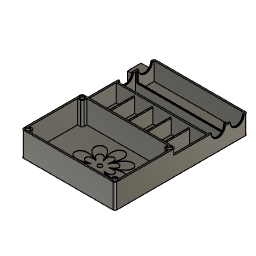
Wingspan - Nectar & Dice Container (Autodesk Fusion 360 design; units mm, degrees)
Autodesk Fusion 360 part; units mm, degrees
note: some values were not read from the file. Set by a fixed rule: which sketch regions a step uses.
sketch "Skizze1" plane through (0, 0, 0) normal (0, 0, 1) x (1, 0, 0)
  line L0 (0, 0) -> (107, 0)
  line L1 (107, 0) -> (107, 152)
  line L2 (107, 152) -> (0, 152)
  line L3 (0, 152) -> (0, 0)
  dimension "d1" = 107
  dimension "d2" = 152
  constraint horizontal L0
  constraint vertical L1
  constraint horizontal L2
  constraint vertical L3
  constraint coincident L0.start L3.end
  measures "d1" distance of L0.start L0.end
  measures "d2" distance of L0.start L2.end
extrude "Extrusion1" add sketch "Skizze1" against normal blind 28
sketch "Skizze2" plane through (0, 0, 0) normal (0, 0, 1) x (-1, 0, 0)
  line L0 (0, -152) -> (0, 0)
  line L1 (0, 0) -> (-107, 0)
  line L2 (-107, 0) -> (-107, -152)
  line L3 (-107, -152) -> (0, -152)
  line L4 (-1.75, -150.25) -> (-105.25, -150.25)
  line L5 (-105.25, -150.25) -> (-105.25, -130.25)
  line L6 (-105.25, -130.25) -> (-1.75, -130.25)
  line L7 (-1.75, -130.25) -> (-1.75, -150.25)
  line L8 (-105.25, -108.5) -> (-1.75, -108.5)
  line L9 (-1.75, -108.5) -> (-1.75, -128.5)
  line L10 (-1.75, -128.5) -> (-105.25, -128.5)
  line L11 (-105.25, -128.5) -> (-105.25, -108.5)
  dimension "d6" = 20
  dimension "d7" = 1.75
  dimension "d8" = 1.75
  dimension "d9" = 1.75
  dimension "d10" = 20
  dimension "d11" = 1.75
  dimension "d12" = 1.75
  dimension "d13" = 1.75
  constraint horizontal L4
  constraint vertical L5
  constraint horizontal L6
  constraint vertical L7
  constraint horizontal L10
  constraint vertical L11
  constraint horizontal L8
  constraint vertical L9
  measures "d6" distance of L4.start L6.end
  measures "d7" distance of L3 L4
  measures "d8" distance of L2 L5
  measures "d9" distance of L0 L7
  measures "d10" distance of L9.end L8.end
  measures "d11" distance of L6 L10
  measures "d12" distance of L2 L11
  measures "d13" distance of L0 L9
extrude "Extrusion2" cut sketch "Skizze2" against normal blind 27 contours L4 L5 L6 L7 | L8 L9 L10 L11
sketch "Skizze3" plane through (0, 0, 0) normal (0, 0, 1) x (-1, 0, 0)
  line L0 (-1.75, -108.5) -> (-1.75, -128.5)
  line L1 (-1.75, -128.5) -> (-105.25, -128.5)
  line L2 (-105.25, -128.5) -> (-105.25, -108.5)
  line L3 (-105.25, -108.5) -> (-1.75, -108.5)
  line L4 (-105.25, -150.25) -> (-105.25, -130.25)
  line L5 (-105.25, -130.25) -> (-1.75, -130.25)
  line L6 (-1.75, -130.25) -> (-1.75, -150.25)
  line L7 (-1.75, -150.25) -> (-105.25, -150.25)
  line L8 (0, -152) -> (0, 0)
  line L9 (0, 0) -> (-107, 0)
  line L10 (-107, 0) -> (-107, -152)
  line L11 (-107, -152) -> (0, -152)
  line L12 (0, -69.5) -> (-107, -69.5)
  dimension "d17" = 82.5
  constraint coincident L8 L12.start
  constraint coincident L10 L12.end
  constraint perpendicular L10 L12
  measures "d17" distance of L11 L12
extrude "Extrusion3" cut sketch "Skizze3" against normal blind 6.5 contours L8 L10 L11 L12
sketch "Skizze4" plane through (0, 0, -6.5) normal (0, 0, 1) x (-1, 0, 0)
  line L0 (-105.25, -128.5) -> (-105.25, -108.5)
  line L1 (-105.25, -108.5) -> (-1.75, -108.5)
  line L2 (-1.75, -108.5) -> (-1.75, -128.5)
  line L3 (-1.75, -128.5) -> (-105.25, -128.5)
  line L4 (-1.75, -130.25) -> (-1.75, -150.25)
  line L5 (-1.75, -150.25) -> (-105.25, -150.25)
  line L6 (-105.25, -150.25) -> (-105.25, -130.25)
  line L7 (-105.25, -130.25) -> (-1.75, -130.25)
  line L8 (0, -69.5) -> (-107, -69.5)
  line L9 (-107, -69.5) -> (-107, -152)
  line L10 (-107, -152) -> (0, -152)
  line L11 (0, -152) -> (0, -69.5)
  line L12 (-1.75, -106.75) -> (-105.25, -106.75)
  line L13 (-105.25, -106.75) -> (-105.25, -71.25)
  line L14 (-105.25, -71.25) -> (-1.75, -71.25)
  line L15 (-1.75, -71.25) -> (-1.75, -106.75)
  dimension "d21" = 1.75
  dimension "d22" = 1.75
  dimension "d23" = 1.75
  dimension "d24" = 1.75
  constraint horizontal L12
  constraint vertical L13
  constraint horizontal L14
  constraint vertical L15
  measures "d21" distance of L1 L12
  measures "d22" distance of L11 L15
  measures "d23" distance of L9 L13
  measures "d24" distance of L8 L14
extrude "Extrusion4" cut sketch "Skizze4" against normal blind 18 contours L12 L13 L14 L15
sketch "Skizze5" plane through (0, 0, -24.5) normal (0, 0, 1) x (-1, 0, 0)
  line L0 (-1.75, -71.25) -> (-105.25, -71.25)
  line L1 (-105.25, -71.25) -> (-105.25, -106.75)
  line L2 (-105.25, -106.75) -> (-1.75, -106.75)
  line L3 (-1.75, -106.75) -> (-1.75, -71.25)
  line L4 (-21.05, -106.75) -> (-22.8, -106.75)
  line L5 (-22.8, -106.75) -> (-22.8, -71.25)
  line L6 (-22.8, -71.25) -> (-21.05, -71.25)
  line L7 (-21.05, -71.25) -> (-21.05, -106.75)
  line L8 (-42.1, -106.75) -> (-43.85, -106.75)
  line L9 (-43.85, -106.75) -> (-43.85, -71.25)
  line L10 (-43.85, -71.25) -> (-42.1, -71.25)
  line L11 (-42.1, -71.25) -> (-42.1, -106.75)
  line L12 (-63.15, -106.75) -> (-64.9, -106.75)
  line L13 (-64.9, -106.75) -> (-64.9, -71.25)
  line L14 (-64.9, -71.25) -> (-63.15, -71.25)
  line L15 (-63.15, -71.25) -> (-63.15, -106.75)
  line L16 (-84.2, -106.75) -> (-85.95, -106.75)
  line L17 (-85.95, -106.75) -> (-85.95, -71.25)
  line L18 (-85.95, -71.25) -> (-84.2, -71.25)
  line L19 (-84.2, -71.25) -> (-84.2, -106.75)
  dimension "d27" = 1.75
  dimension "d28" = 1.75
  dimension "d29" = 1.75
  dimension "d30" = 1.75
  dimension "d31" = 19.3
  dimension "d32" = 19.3
  dimension "d33" = 19.3
  dimension "d34" = 19.3
  constraint horizontal L4
  constraint vertical L5
  constraint horizontal L6
  constraint vertical L7
  constraint coincident L0 L5.end
  constraint coincident L2 L4.start
  constraint horizontal L8
  constraint vertical L9
  constraint horizontal L10
  constraint vertical L11
  constraint coincident L0 L9.end
  constraint coincident L2 L8.start
  constraint horizontal L12
  constraint vertical L13
  constraint horizontal L14
  constraint vertical L15
  constraint coincident L0 L13.end
  constraint horizontal L16
  constraint vertical L17
  constraint horizontal L18
  constraint vertical L19
  constraint coincident L0 L17.end
  constraint coincident L2 L16.start
  measures "d27" distance of L5 L7
  measures "d28" distance of L9 L11
  measures "d29" distance of L13 L15
  measures "d30" distance of L17 L19
  measures "d31" distance of L3 L7
  measures "d32" distance of L5 L11
  measures "d33" distance of L9 L15
  measures "d34" distance of L13 L19
extrude "Extrusion5" add sketch "Skizze5" along normal blind 15 contours L0 L2 L4 L5 L6 L7 | L0 L2 L8 L9 L10 L11 | L0 L2 L12 L13 L14 L15 | L0 L2 L16 L17 L18 L19
sketch "Skizze6" plane through (0, 0, 0) normal (0, 0, 1) x (-1, 0, 0)
  line L0 (-107, -69.5) -> (0, -69.5)
  line L1 (0, -69.5) -> (0, 0)
  line L2 (0, 0) -> (-107, 0)
  line L3 (-107, 0) -> (-107, -69.5)
  line L4 (0, -69.5) -> (-7, -69.5)
  line L5 (-7, -69.5) -> (-7, -62.5)
  line L6 (-7, -62.5) -> (0, -62.5)
  line L7 (0, -62.5) -> (0, -69.5)
  line L8 (-107, -69.5) -> (-100, -69.5)
  line L9 (-100, -69.5) -> (-100, -62.5)
  line L10 (-100, -62.5) -> (-107, -62.5)
  line L11 (-107, -62.5) -> (-107, -69.5)
  line L12 (-107, 0) -> (-100, 0)
  line L13 (-100, 0) -> (-100, -7)
  line L14 (-100, -7) -> (-107, -7)
  line L15 (-107, -7) -> (-107, 0)
  line L16 (0, 0) -> (-7, 0)
  line L17 (-7, 0) -> (-7, -7)
  line L18 (-7, -7) -> (0, -7)
  line L19 (0, -7) -> (0, 0)
  circle A0 centre (-3.5, -3.5) radius 2.65
  circle A1 centre (-103.5, -3.5) radius 2.65
  circle A2 centre (-103.5, -66) radius 2.65
  circle A3 centre (-3.5, -66) radius 2.65
  line L20 (-7, -67.75) -> (-100, -67.75)
  line L21 (-100, -67.75) -> (-100, -1.75)
  line L22 (-100, -1.75) -> (-7, -1.75)
  line L23 (-7, -1.75) -> (-7, -67.75)
  line L24 (-7, -62.5) -> (-1.75, -62.5)
  line L25 (-1.75, -62.5) -> (-1.75, -7)
  line L26 (-1.75, -7) -> (-7, -7)
  line L27 (-7, -7) -> (-7, -62.5)
  line L28 (-100, -7) -> (-105.25, -7)
  line L29 (-105.25, -7) -> (-105.25, -62.5)
  line L30 (-105.25, -62.5) -> (-100, -62.5)
  line L31 (-100, -62.5) -> (-100, -7)
  dimension "d37" = 7
  dimension "d38" = 7
  dimension "d39" = 7
  dimension "d40" = 7
  dimension "d41" = 7
  dimension "d42" = 7
  dimension "d43" = 7
  dimension "d44" = 7
  dimension "d45" = 5.3
  dimension "d46" = 5.3
  dimension "d47" = 5.3
  dimension "d48" = 5.3
  dimension "d49" = 3.5
  dimension "d50" = 3.5
  dimension "d51" = 3.5
  dimension "d52" = 3.5
  dimension "d53" = 3.5
  dimension "d54" = 3.5
  dimension "d55" = 3.5
  dimension "d56" = 3.5
  dimension "d57" = 1.75
  dimension "d58" = 1.75
  dimension "d59" = 7
  dimension "d60" = 7
  dimension "d61" = 1.75
  dimension "d62" = 1.75
  constraint horizontal L4
  constraint vertical L5
  constraint horizontal L6
  constraint vertical L7
  constraint coincident L0.end L1.start
  constraint horizontal L8
  constraint vertical L9
  constraint horizontal L10
  constraint vertical L11
  constraint coincident L0.start L3.end
  constraint horizontal L12
  constraint vertical L13
  constraint horizontal L14
  constraint vertical L15
  constraint coincident L2.end L3.start
  constraint horizontal L16
  constraint vertical L17
  constraint horizontal L18
  constraint vertical L19
  constraint coincident L1.end L2.start
  constraint horizontal L20
  constraint vertical L21
  constraint horizontal L22
  constraint vertical L23
  constraint horizontal L24
  constraint vertical L25
  constraint horizontal L26
  constraint vertical L27
  constraint coincident L18 L25.end
  constraint horizontal L28
  constraint vertical L29
  constraint horizontal L30
  constraint vertical L31
  constraint coincident L10 L29.end
  measures "d37" distance of L0.end L4.end
  measures "d38" distance of L0.end L6.end
  measures "d39" distance of L0.start L8.end
  measures "d40" distance of L0.start L10.end
  measures "d41" distance of L2.end L12.end
  measures "d42" distance of L2.end L14.end
  measures "d43" distance of L1.end L16.end
  measures "d44" distance of L1.end L18.end
  measures "d45" diameter of A0
  measures "d46" diameter of A1
  measures "d47" diameter of A2
  measures "d48" diameter of A3
  measures "d49" distance of L7 A3.centre
  measures "d50" distance of L6 A3.centre
  measures "d51" distance of L10 A2.centre
  measures "d52" distance of L11 A2.centre
  measures "d53" distance of L15 A1.centre
  measures "d54" distance of L14 A1.centre
  measures "d55" distance of L18 A0.centre
  measures "d56" distance of L17 A0.centre
  measures "d57" distance of L0 L20
  measures "d58" distance of L2 L22
  measures "d59" distance of L1 L23
  measures "d60" distance of L3 L21
  measures "d61" distance of L1 L25
  measures "d62" distance of L3 L29
extrude "Extrusion6" cut sketch "Skizze6" against normal blind 26.25 contours L5 L9 L13 L17 L20 L21 L22 L23 L27 L31 | L10 L14 L21 L28 L29 L30 L31 | L6 L18 L23 L24 L25 L26 L27
extrude "Extrusion7" cut sketch "Skizze6" against normal blind 1.2 contours A0 | A1 | A2 | A3
sketch "Skizze7" plane through (0, 0, 0) normal (-1, 0, 0) x (0, -1, 0)
  line L0 (-69.5, 0) -> (-69.5, -6.5)
  line L1 (-69.5, -6.5) -> (-152, -6.5)
  line L2 (-152, -6.5) -> (-152, -28)
  line L3 (-152, -28) -> (0, -28)
  line L4 (0, -28) -> (0, 0)
  line L5 (0, 0) -> (-69.5, 0)
  line L6 (-152, -28) -> (-136.5, -28)
  line L7 (-136.5, -28) -> (-136.5, -18)
  line L8 (-136.5, -18) -> (-152, -18)
  line L9 (-152, -18) -> (-152, -28)
  dimension "d67" = 15.5
  dimension "d68" = 10
  constraint horizontal L6
  constraint vertical L7
  constraint horizontal L8
  constraint vertical L9
  constraint coincident L2.end L3.start
  measures "d67" distance of L2.end L6.end
  measures "d68" distance of L2.end L8.end
extrude "Extrusion8" add sketch "Skizze7" along normal blind 10 contours L2 L3 L6 L7 L8 L9
sketch "Skizze8" plane through (107, 0, 0) normal (1, 0, 0) x (0, 1, 0)
  line L0 (69.5, -6.5) -> (69.5, 0)
  line L1 (69.5, 0) -> (0, 0)
  line L2 (0, 0) -> (0, -28)
  line L3 (0, -28) -> (152, -28)
  line L4 (152, -28) -> (152, -6.5)
  line L5 (152, -6.5) -> (69.5, -6.5)
  circle A0 centre (140.25, -6.5) radius 7.5
  circle A1 centre (118.5, -6.5) radius 7.5
  dimension "d71" = 15
  dimension "d72" = 11.75
  dimension "d73" = 15
  dimension "d74" = 21.75
  constraint coincident L5 A0.centre
  constraint coincident L5 A1.centre
  measures "d71" diameter of A0
  measures "d72" distance of L4.end A0.centre
  measures "d73" diameter of A1
  measures "d74" distance of A0.centre A1.centre
extrude "Extrusion9" cut sketch "Skizze8" against normal blind 145 contours L5 A1 | L5 A0 picked at (120.0587, -9.1998) picked at (142.75, -10.4092)
extrude "Extrusion10" cut 1 faces at (-10, 146.8333, -24.6667) along direction (1, 0, 0) blind 10
sketch "Skizze9" plane through (0, 0, -6.5) normal (0, 0, 1) x (-1, 0, 0)
  line L0 (-107, -132.75) -> (-105.25, -132.75)
  line L1 (-105.25, -132.75) -> (-105.25, -130.25)
  line L2 (-105.25, -130.25) -> (-1.75, -130.25)
  line L3 (-1.75, -130.25) -> (-1.75, -132.75)
  line L4 (-1.75, -132.75) -> (0, -132.75)
  line L5 (0, -132.75) -> (0, -126)
  line L6 (0, -126) -> (-1.75, -126)
  line L7 (-1.75, -126) -> (-1.75, -128.5)
  line L8 (-1.75, -128.5) -> (-105.25, -128.5)
  line L9 (-105.25, -128.5) -> (-105.25, -126)
  line L10 (-105.25, -126) -> (-107, -126)
  line L11 (-107, -126) -> (-107, -132.75)
  line L12 (-4, -130.25) -> (-103, -130.25)
  line L13 (-103, -130.25) -> (-103, -128.5)
  line L14 (-103, -128.5) -> (-4, -128.5)
  line L15 (-4, -128.5) -> (-4, -130.25)
  dimension "d79" = 4
  dimension "d80" = 4
  constraint horizontal L12
  constraint vertical L13
  constraint horizontal L14
  constraint vertical L15
  constraint coincident L8 L13.end
  constraint coincident L2 L12.start
  measures "d79" distance of L5 L15
  measures "d80" distance of L11 L13
extrude "Extrusion11" cut sketch "Skizze9" against normal blind 10 contours L2 L8 L12 L13 L14 L15
extrude "Extrusion12" add sketch "Skizze7" along normal blind 15 contours L2 L3 L6 L7 L8 L9
fillet "Abrundung1" radius 2 6 edges at (0, 0, -14) (107, 0, -14) (7, 62.5, -13.125) (100, 62.5, -13.125) (100, 7, -13.125) (7, 7, -13.125)
fillet "Abrundung2" radius 2 2 edges at (107, 69.5, -3.25) (0, 69.5, -3.25)
fillet "Abrundung3" radius 2 2 edges at (107, 152, -17.25) (0, 152, -12.25)
fillet "Abrundung4" radius 0.5 2 edges at (53.5, 130.25, -16.5) (53.5, 128.5, -16.5)
fillet "Abrundung5" radius 0.75 8 edges at (22.8, 89, -9.5) (21.05, 89, -9.5) (43.85, 89, -9.5) (42.1, 89, -9.5) (64.9, 89, -9.5) (63.15, 89, -9.5) (85.95, 89, -9.5) (84.2, 89, -9.5)
sketch "Skizze10" plane through (0, 0, -26.25) normal (0, 0, 1) x (-1, 0, 0)
  line L0 (-102, -7) -> (-105.25, -7)
  line L1 (-105.25, -7) -> (-105.25, -62.5)
  line L2 (-105.25, -62.5) -> (-102, -62.5)
  arc A0 (-100, -64.5) -> (-102, -62.5) centre (-102, -64.5) ccw
  line L3 (-100, -64.5) -> (-100, -67.75)
  line L4 (-100, -67.75) -> (-7, -67.75)
  line L5 (-7, -67.75) -> (-7, -64.5)
  arc A1 (-5, -62.5) -> (-7, -64.5) centre (-5, -64.5) ccw
  line L6 (-5, -62.5) -> (-1.75, -62.5)
  line L7 (-1.75, -62.5) -> (-1.75, -7)
  line L8 (-1.75, -7) -> (-5, -7)
  arc A2 (-7, -5) -> (-5, -7) centre (-5, -5) ccw
  line L9 (-7, -5) -> (-7, -1.75)
  line L10 (-7, -1.75) -> (-100, -1.75)
  line L11 (-100, -1.75) -> (-100, -5)
  arc A3 (-102, -7) -> (-100, -5) centre (-102, -5) ccw
  spline S0 degree 3 poles (-56.5592, -62.8702) (-58.3493, -62.3021) (-60.0393, -60.5207) (-60.7133, -58.4915) knots 0 0 0 0 1 1 1 1
  spline S1 degree 3 poles (-60.7133, -58.4915) (-61.4989, -56.1264) (-61.1983, -52.2556) (-59.8935, -47.9352) knots 0 0 0 0 1 1 1 1
  spline S2 degree 3 poles (-59.8935, -47.9352) (-59.3339, -46.082) (-58.9465, -44.4517) (-59.0327, -44.3123) knots 0 0 0 0 1 1 1 1
  spline S3 degree 3 poles (-59.0327, -44.3123) (-59.1188, -44.1728) (-58.7988, -43.3306) (-58.3216, -42.4407) knots 0 0 0 0 1 1 1 1
  spline S4 degree 3 poles (-58.3216, -42.4407) (-57.8443, -41.5508) (-57.5275, -41.1269) (-57.6175, -41.4989) knots 0 0 0 0 1 1 1 1
  spline S5 degree 3 poles (-57.6175, -41.4989) (-57.7075, -41.8708) (-57.9588, -42.9002) (-58.176, -43.7864) knots 0 0 0 0 1 1 1 1
  spline S6 degree 3 poles (-58.176, -43.7864) (-58.3931, -44.6726) (-58.4995, -46.2578) (-58.4123, -47.309) knots 0 0 0 0 1 1 1 1
  spline S7 degree 3 poles (-58.4123, -47.309) (-58.2782, -48.9263) (-58.0889, -49.3677) (-57.1821, -50.178) knots 0 0 0 0 1 1 1 1
  spline S8 degree 3 poles (-57.1821, -50.178) (-55.6542, -51.5432) (-54.0418, -51.4908) (-52.5795, -50.0285) knots 0 0 0 0 1 1 1 1
  spline S9 degree 3 poles (-52.5795, -50.0285) (-50.8387, -48.2877) (-50.7558, -45.8848) (-52.2827, -41.4252) knots 0 0 0 0 1 1 1 1
  spline S10 degree 3 poles (-52.2827, -41.4252) (-52.3962, -41.0938) (-51.8778, -41.8116) (-51.1307, -43.0205) knots 0 0 0 0 1 1 1 1
  spline S11 degree 3 poles (-51.1307, -43.0205) (-49.292, -45.9958) (-47.7092, -47.2471) (-45.7844, -47.2471) knots 0 0 0 0 1 1 1 1
  spline S12 degree 3 poles (-45.7844, -47.2471) (-44.615, -47.2471) (-44.1039, -47.049) (-43.3644, -46.3095) knots 0 0 0 0 1 1 1 1
  spline S13 degree 3 poles (-43.3644, -46.3095) (-41.3829, -44.328) (-42.4992, -41.0532) (-45.8196, -39.1074) knots 0 0 0 0 1 1 1 1
  spline S14 degree 3 poles (-45.8196, -39.1074) (-47.2511, -38.2685) (-47.7575, -37.6104) (-46.9716, -37.6104) knots 0 0 0 0 1 1 1 1
  spline S15 degree 3 poles (-46.9716, -37.6104) (-46.7747, -37.6104) (-46.6847, -37.7256) (-46.7717, -37.8663) knots 0 0 0 0 1 1 1 1
  spline S16 degree 3 poles (-46.7717, -37.8663) (-46.8587, -38.0071) (-45.801, -38.1656) (-44.4211, -38.2186) knots 0 0 0 0 1 1 1 1
  spline S17 degree 3 poles (-44.4211, -38.2186) (-41.4525, -38.3326) (-39.7946, -37.7064) (-39.0007, -36.1712) knots 0 0 0 0 1 1 1 1
  spline S18 degree 3 poles (-39.0007, -36.1712) (-37.9053, -34.053) (-39.4569, -31.4883) (-42.138, -30.9853) knots 0 0 0 0 1 1 1 1
  spline S19 degree 3 poles (-42.138, -30.9853) (-43.1628, -30.7931) (-45.7249, -31.1569) (-47.6678, -31.7705) knots 0 0 0 0 1 1 1 1
  spline S20 degree 3 poles (-47.6678, -31.7705) (-47.9468, -31.8586) (-47.2483, -31.3259) (-46.1157, -30.5867) knots 0 0 0 0 1 1 1 1
  spline S21 degree 3 poles (-46.1157, -30.5867) (-43.7478, -29.0412) (-42.5959, -27.4189) (-42.5959, -25.6292) knots 0 0 0 0 1 1 1 1
  spline S22 degree 3 poles (-42.5959, -25.6292) (-42.5959, -23.9375) (-43.1044, -23.1064) (-44.4952, -22.5253) knots 0 0 0 0 1 1 1 1
  spline S23 degree 3 poles (-44.4952, -22.5253) (-46.2045, -21.8111) (-47.9424, -22.3756) (-49.568, -24.173) knots 0 0 0 0 1 1 1 1
  spline S24 degree 3 poles (-49.568, -24.173) (-50.2812, -24.9616) (-50.9936, -25.565) (-51.1511, -25.5139) knots 0 0 0 0 1 1 1 1
  spline S25 degree 3 poles (-51.1511, -25.5139) (-51.3086, -25.4628) (-51.3439, -25.5725) (-51.2295, -25.7576) knots 0 0 0 0 1 1 1 1
  spline S26 degree 3 poles (-51.2295, -25.7576) (-51.021, -26.0949) (-51.9974, -28.3217) (-52.2451, -28.0739) knots 0 0 0 0 1 1 1 1
  spline S27 degree 3 poles (-52.2451, -28.0739) (-52.3176, -28.0015) (-52.1542, -27.2023) (-51.882, -26.2981) knots 0 0 0 0 1 1 1 1
  spline S28 degree 3 poles (-51.882, -26.2981) (-50.8258, -22.7886) (-51.5141, -19.8497) (-53.6271, -18.847) knots 0 0 0 0 1 1 1 1
  spline S29 degree 3 poles (-53.6271, -18.847) (-55.6301, -17.8965) (-57.5857, -18.8268) (-58.4654, -21.1486) knots 0 0 0 0 1 1 1 1
  spline S30 degree 3 poles (-58.4654, -21.1486) (-59.0459, -22.6806) (-58.7942, -24.8474) (-57.6334, -28.3119) knots 0 0 0 0 1 1 1 1
  spline S31 degree 3 poles (-57.6334, -28.3119) (-57.5088, -28.6838) (-57.8962, -28.1512) (-58.4944, -27.1284) knots 0 0 0 0 1 1 1 1
  spline S32 degree 3 poles (-58.4944, -27.1284) (-60.4538, -23.778) (-62.1707, -22.3946) (-64.3696, -22.3946) knots 0 0 0 0 1 1 1 1
  spline S33 degree 3 poles (-64.3696, -22.3946) (-68.1521, -22.3946) (-68.6377, -27.3285) (-65.1088, -29.9052) knots 0 0 0 0 1 1 1 1
  spline S34 degree 3 poles (-65.1088, -29.9052) (-64.3499, -30.4593) (-63.7732, -31.0689) (-63.8273, -31.2599) knots 0 0 0 0 1 1 1 1
  spline S35 degree 3 poles (-63.8273, -31.2599) (-63.8847, -31.4625) (-63.6735, -31.511) (-63.3201, -31.3765) knots 0 0 0 0 1 1 1 1
  spline S36 degree 3 poles (-63.3201, -31.3765) (-62.9224, -31.225) (-62.8306, -31.2596) (-63.0527, -31.4773) knots 0 0 0 0 1 1 1 1
  spline S37 degree 3 poles (-63.0527, -31.4773) (-63.2735, -31.6937) (-63.983, -31.6897) (-65.098, -31.4659) knots 0 0 0 0 1 1 1 1
  spline S38 degree 3 poles (-65.098, -31.4659) (-68.378, -30.8075) (-71.3368, -32.4955) (-71.3368, -35.0251) knots 0 0 0 0 1 1 1 1
  spline S39 degree 3 poles (-71.3368, -35.0251) (-71.3368, -38.0388) (-67.7534, -39.4474) (-63.4113, -38.1407) knots 0 0 0 0 1 1 1 1
  spline S40 degree 3 poles (-63.4113, -38.1407) (-61.5097, -37.5684) (-61.5064, -37.5632) (-64.1235, -39.2548) knots 0 0 0 0 1 1 1 1
  spline S41 degree 3 poles (-64.1235, -39.2548) (-67.6237, -41.5171) (-68.5135, -44.6269) (-66.2141, -46.5617) knots 0 0 0 0 1 1 1 1
  spline S42 degree 3 poles (-66.2141, -46.5617) (-64.4839, -48.0175) (-61.8719, -47.4084) (-59.9372, -45.0979) knots 0 0 0 0 1 1 1 1
  spline S43 degree 3 poles (-59.9372, -45.0979) (-59.5254, -44.6062) (-59.1831, -44.3384) (-59.1764, -44.5028) knots 0 0 0 0 1 1 1 1
  spline S44 degree 3 poles (-59.1764, -44.5028) (-59.1603, -44.8983) (-61.7652, -50.0133) (-62.6404, -51.3046) knots 0 0 0 0 1 1 1 1
  spline S45 degree 3 poles (-62.6404, -51.3046) (-64.8787, -54.6074) (-67.8698, -56.5364) (-70.7619, -56.5423) knots 0 0 0 0 1 1 1 1
  spline S46 degree 3 poles (-70.7619, -56.5423) (-74.6622, -56.5503) (-77.4468, -52.9616) (-76.4404, -49.2242) knots 0 0 0 0 1 1 1 1
  spline S47 degree 3 poles (-76.4404, -49.2242) (-75.5977, -46.0946) (-73.3487, -43.7833) (-68.2937, -40.8517) knots 0 0 0 0 1 1 1 1
  spline S48 degree 3 poles (-68.2937, -40.8517) (-67.0849, -40.1506) (-66.4002, -39.6772) (-66.7721, -39.7996) knots 0 0 0 0 1 1 1 1
  spline S49 degree 3 poles (-66.7721, -39.7996) (-69.2344, -40.6101) (-74.0069, -41.6679) (-75.201, -41.6679) knots 0 0 0 0 1 1 1 1
  spline S50 degree 3 poles (-75.201, -41.6679) (-78.3788, -41.6679) (-81.566, -40.0721) (-82.6763, -37.925) knots 0 0 0 0 1 1 1 1
  spline S51 degree 3 poles (-82.6763, -37.925) (-83.3903, -36.5444) (-83.3099, -33.6152) (-82.5226, -32.324) knots 0 0 0 0 1 1 1 1
  spline S52 degree 3 poles (-82.5226, -32.324) (-81.7029, -30.9798) (-79.9968, -29.6996) (-78.2996, -29.1552) knots 0 0 0 0 1 1 1 1
  spline S53 degree 3 poles (-78.2996, -29.1552) (-76.383, -28.5404) (-71.7514, -28.9223) (-68.2937, -29.9801) knots 0 0 0 0 1 1 1 1
  spline S54 degree 3 poles (-68.2937, -29.9801) (-66.7129, -30.4637) (-65.1153, -30.9414) (-64.7433, -31.0416) knots 0 0 0 0 1 1 1 1
  spline S55 degree 3 poles (-64.7433, -31.0416) (-64.3714, -31.1419) (-65.6092, -30.4005) (-67.4941, -29.3941) knots 0 0 0 0 1 1 1 1
  spline S56 degree 3 poles (-67.4941, -29.3941) (-72.2017, -26.8806) (-73.8514, -25.6231) (-75.3197, -23.4291) knots 0 0 0 0 1 1 1 1
  spline S57 degree 3 poles (-75.3197, -23.4291) (-76.4762, -21.7011) (-76.5778, -21.356) (-76.5778, -19.1561) knots 0 0 0 0 1 1 1 1
  spline S58 degree 3 poles (-76.5778, -19.1561) (-76.5778, -17.0784) (-76.4577, -16.6054) (-75.6671, -15.5688) knots 0 0 0 0 1 1 1 1
  spline S59 degree 3 poles (-75.6671, -15.5688) (-73.5767, -12.8281) (-69.7646, -12.4778) (-66.4998, -14.7263) knots 0 0 0 0 1 1 1 1
  spline S60 degree 3 poles (-66.4998, -14.7263) (-64.4837, -16.1149) (-63.2894, -17.6345) (-60.7914, -21.9893) knots 0 0 0 0 1 1 1 1
  spline S61 degree 3 poles (-60.7914, -21.9893) (-59.8635, -23.607) (-59.1786, -24.6915) (-59.2695, -24.3993) knots 0 0 0 0 1 1 1 1
  spline S62 degree 3 poles (-59.2695, -24.3993) (-59.3604, -24.1071) (-59.8438, -22.5855) (-60.3437, -21.018) knots 0 0 0 0 1 1 1 1
  spline S63 degree 3 poles (-60.3437, -21.018) (-61.4281, -17.6182) (-61.7986, -13.6027) (-61.2022, -11.7145) knots 0 0 0 0 1 1 1 1
  spline S64 degree 3 poles (-61.2022, -11.7145) (-59.817, -7.3289) (-55.9762, -5.3552) (-52.3885, -7.1855) knots 0 0 0 0 1 1 1 1
  spline S65 degree 3 poles (-52.3885, -7.1855) (-48.7171, -9.0585) (-47.7733, -14.2699) (-49.879, -21.0421) knots 0 0 0 0 1 1 1 1
  spline S66 degree 3 poles (-49.879, -21.0421) (-51.2433, -25.4298) (-51.2167, -25.5019) (-49.4657, -22.1589) knots 0 0 0 0 1 1 1 1
  spline S67 degree 3 poles (-49.4657, -22.1589) (-47.2727, -17.9721) (-45.9857, -16.2284) (-44.052, -14.8244) knots 0 0 0 0 1 1 1 1
  spline S68 degree 3 poles (-44.052, -14.8244) (-41.0966, -12.6788) (-38.3228, -12.4229) (-35.8388, -14.0667) knots 0 0 0 0 1 1 1 1
  spline S69 degree 3 poles (-35.8388, -14.0667) (-32.6466, -16.1792) (-32.583, -20.6998) (-35.6935, -24.3965) knots 0 0 0 0 1 1 1 1
  spline S70 degree 3 poles (-35.6935, -24.3965) (-36.7851, -25.6938) (-39.6299, -27.663) (-42.5114, -29.1158) knots 0 0 0 0 1 1 1 1
  spline S71 degree 3 poles (-42.5114, -29.1158) (-43.6737, -29.7018) (-44.6247, -30.2455) (-44.6247, -30.3241) knots 0 0 0 0 1 1 1 1
  spline S72 degree 3 poles (-44.6247, -30.3241) (-44.6247, -30.4026) (-43.2933, -30.0073) (-41.6661, -29.4456) knots 0 0 0 0 1 1 1 1
  spline S73 degree 3 poles (-41.6661, -29.4456) (-37.8603, -28.132) (-33.6642, -27.7981) (-31.2092, -28.6136) knots 0 0 0 0 1 1 1 1
  spline S74 degree 3 poles (-31.2092, -28.6136) (-25.6033, -30.4756) (-25.0764, -37.2838) (-30.3383, -39.8677) knots 0 0 0 0 1 1 1 1
  spline S75 degree 3 poles (-30.3383, -39.8677) (-33.0905, -41.2191) (-36.6516, -41.1596) (-41.4863, -39.6813) knots 0 0 0 0 1 1 1 1
  spline S76 degree 3 poles (-41.4863, -39.6813) (-43.3866, -39.1002) (-45.0603, -38.6277) (-45.2057, -38.6313) knots 0 0 0 0 1 1 1 1
  spline S77 degree 3 poles (-45.2057, -38.6313) (-45.3511, -38.6349) (-44.0838, -39.3737) (-42.3896, -40.2731) knots 0 0 0 0 1 1 1 1
  spline S78 degree 3 poles (-42.3896, -40.2731) (-36.727, -43.2794) (-35.2415, -44.5962) (-33.7765, -47.9079) knots 0 0 0 0 1 1 1 1
  spline S79 degree 3 poles (-33.7765, -47.9079) (-31.8468, -52.2705) (-35.0863, -56.9686) (-39.6514, -56.4279) knots 0 0 0 0 1 1 1 1
  spline S80 degree 3 poles (-39.6514, -56.4279) (-43.0487, -56.0255) (-45.9001, -53.4633) (-48.9635, -48.0601) knots 0 0 0 0 1 1 1 1
  spline S81 degree 3 poles (-48.9635, -48.0601) (-49.9551, -46.3111) (-50.6671, -45.1845) (-50.5457, -45.5564) knots 0 0 0 0 1 1 1 1
  spline S82 degree 3 poles (-50.5457, -45.5564) (-49.4838, -48.8096) (-48.6148, -52.3281) (-48.4531, -54.0293) knots 0 0 0 0 1 1 1 1
  spline S83 degree 3 poles (-48.4531, -54.0293) (-47.8919, -59.9342) (-51.9307, -64.3391) (-56.5592, -62.8702) knots 0 0 0 0 1 1 1 1
  spline S84 degree 3 poles (-48.3441, -37.6104) (-48.7775, -37.3303) (-48.7652, -37.2819) (-48.2595, -37.2774) knots 0 0 0 0 1 1 1 1
  spline S85 degree 3 poles (-48.2595, -37.2774) (-47.9341, -37.2748) (-47.6678, -37.4244) (-47.6678, -37.6104) knots 0 0 0 0 1 1 1 1
  spline S86 degree 3 poles (-47.6678, -37.6104) (-47.6678, -38.0228) (-47.706, -38.0228) (-48.3441, -37.6104) knots 0 0 0 0 1 1 1 1
  spline S87 degree 3 poles (-56.6436, -36.4423) (-58.0914, -34.9945) (-57.4186, -32.8343) (-55.3688, -32.3493) knots 0 0 0 0 1 1 1 1
  spline S88 degree 3 poles (-55.3688, -32.3493) (-54.6302, -32.1746) (-54.2445, -32.3343) (-53.4245, -33.1542) knots 0 0 0 0 1 1 1 1
  spline S89 degree 3 poles (-53.4245, -33.1542) (-52.8619, -33.7168) (-52.4016, -34.5) (-52.4016, -34.8947) knots 0 0 0 0 1 1 1 1
  spline S90 degree 3 poles (-52.4016, -34.8947) (-52.4016, -35.8869) (-53.8793, -37.2723) (-54.9376, -37.2723) knots 0 0 0 0 1 1 1 1
  spline S91 degree 3 poles (-54.9376, -37.2723) (-55.4194, -37.2723) (-56.1871, -36.8988) (-56.6436, -36.4423) knots 0 0 0 0 1 1 1 1
  spline S92 degree 3 poles (-62.7237, -31.877) (-62.6138, -31.6991) (-62.3005, -31.6393) (-62.0275, -31.7441) knots 0 0 0 0 1 1 1 1
  spline S93 degree 3 poles (-62.0275, -31.7441) (-61.3285, -32.0123) (-61.4109, -32.2003) (-62.2273, -32.2003) knots 0 0 0 0 1 1 1 1
  spline S94 degree 3 poles (-62.2273, -32.2003) (-62.6102, -32.2003) (-62.8336, -32.0548) (-62.7237, -31.877) knots 0 0 0 0 1 1 1 1
extrude "Extrusion13" cut sketch "Skizze10" against normal blind 0.4 contours S0 S1 S2 S3 S4 S5 S6 S7 S8 S9 S10 S11 S12 S13 S14 S15 S16 S17 S18 S19 S20 S21 S22 S23 S24 S25 S26 S27 S28 S29 S30 S31 S32 S33 S34 S35 S36 S37 S38 S39 S40 S41 S42 S43 S44 S45 S46 S47 S48 S49 S50 S51 S52 S53 S54 S55 S56 S57 S58 S59 S60 S61 S62 S63 S64 S65 S66 S67 S68 S69 S70 S71 S72 S73 S74 S75 S76 S77 S78 S79 S80 S81 S82 S83 | S87 S88 S89 S90 S91
fillet "Abrundung6" radius 0.5 2 edges at (103, 130.25, -11.75) (103, 128.5, -11.75)
fillet "Abrundung7" radius 0.5 2 edges at (4, 128.5, -11.75) (4, 130.25, -11.75)
fillet "Abrundung8" radius 0.5 4 edges at (0, 140.25, -14) (0, 118.5, -14) (1.75, 118.5, -14) (1.75, 140.25, -14)
fillet "Abrundung9" radius 0.5 4 edges at (105.25, 118.5, -14) (105.25, 140.25, -14) (107, 140.25, -14) (107, 118.5, -14)
extrude "Extrusion14" cut 5 faces at (92.3833, 94.9167, -24.5) (71.3333, 83.0833, -24.5) (50.2833, 83.0833, -24.5) (29.2333, 94.9167, -24.5) (14.6167, 83.0833, -24.5) along direction (0, 0, -1) blind 2
extrude "Extrusion15" cut 1 faces at (36.8333, 130.25, -23.6667) along direction (0, -1, 0) blind 0.4
extrude "Extrusion16" cut 1 faces at (70.1667, 128.5, -23.6667) along direction (0, 1, 0) blind 0.4
equation "d14 = -28 mm + 1 mm"
equation "d63 = -28 mm + 1.75 mm"
equation "d72 = 10 mm + 1.75 mm"
equation "d74 = 20 mm + 1.75 mm"
